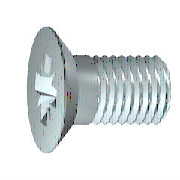
# Autodesk Inventor part: NF EN ISO 7046-2 H - M3x4 - 8.8 - H1
Saved by Autodesk Inventor 2019 (Build 230136000, 136)
## iProperties
Created: 2018-01-05
Part Number: NF EN ISO 7046-2 H - M3x4 - 8.8 - H1
Material: Acier inoxydable 440C
Description: Vis à tête fraisée plate (type de tête standard) avec empreinte cruciforme de type H ou Z
Document SubType Name: Modeling
Standard: NF EN ISO 7046-2 H
Designer: Sébastien DI MERCURIO
Standards Organization: AFNOR
Language: fr-FR
Size Designation: M3x4 - 8.8 - H1
Categories: <MemberInstance><Categories><Category DisplayName="Visserie" InternalName="e4da775c-781d-43d5-af7c-5136215cf5a6" Mnemonic="FSTN"><Category DisplayName="Vis" InternalName="536e6df0-f778-49ac-b2f2-25c71d2aa0b2" Mnemonic="SCRW"><CategoryParameter DisplayName="Désignation du diamètre nominal" InternalName="03caf894-eafd-4c09-a035-916ac084b87b" Mnemonic="nomdiadesig"/><CategoryParameter DisplayName="Longueur nominale" InternalName="238ecbaf-3e6c-45dd-aa95-4068c8e0fd02" Mnemonic="nomlen"/><CategoryParameter DisplayName="Désignation du filetage" InternalName="586d5e89-370a-4089-914f-0110033585c7" Mnemonic="thrdesign"/><CategoryParameter DisplayName="Désignation de série de filetage" InternalName="87c5849c-b3a5-4c3e-9c9b-2feecef9be86" Mnemonic="thrserdsgn"/><CategoryParameter DisplayName="Diamètre nominal" InternalName="8bbe3f8e-44cf-40a9-a251-3a6edc8168d6" Mnemonic="nomdia"/><CategoryParameter DisplayName="Type de taraudage" InternalName="b4bbb7bc-d6aa-4c9f-a9a9-4152b9f6fe49" Mnemonic="thrtype"/><CategoryParameter DisplayName="Pas de filetage" InternalName="bb82302e-82d8-4176-8fc1-c5d7bb17d5ad" Mnemonic="pitch1"/><CategoryParameter DisplayName="Filets par unité" InternalName="bdc6e7d2-ffd0-4d9c-a173-16b95ebb912d" Mnemonic="thrperunit1"/><CategoryParameter DisplayName="Classe de filetage" InternalName="ebc0d23b-2cc6-4d2a-b376-d52aae53bab6" Mnemonic="thrclss"/><Category DisplayName="Tête fraisée" InternalName="49656530-5684-4604-a233-68d537625f23" Mnemonic="CSSCRW"><CategoryParameter DisplayName="Type" InternalName="161b33bb-bee3-4fab-a17d-97511dff40f0" Mnemonic="type"/><CategoryParameter DisplayName="Longueur de filetage" InternalName="207f0278-6dec-43ab-bffc-1c6d03e64de4" Mnemonic="thrlen"/><CategoryParameter DisplayName="Longueur de serrage" InternalName="2fff3de5-ce2a-45fd-9425-99ddc9dff352" Mnemonic="grplen"/><CategoryParameter DisplayName="Classe de propriétés" InternalName="5249b721-5ecc-4781-a2e8-d7e3bda3ecca" Mnemonic="propclss"/><CategoryParameter DisplayName="Hauteur de tête" InternalName="57526df9-da71-45fb-acb4-1d0529a34778" Mnemonic="headh"/><CategoryParameter DisplayName="Diamètre de tige" InternalName="7ece923f-d8ee-40d5-83f8-980cad520964" Mnemonic="grpdia"/><CategoryParameter DisplayName="Diamètre de tête" InternalName="a509cd31-06d1-44c5-b54e-d7a695352906" Mnemonic="headdia"/><CategoryParameter DisplayName="Angle de tête" InternalName="dbcfc1e0-7990-403e-bc2e-90d1c639222a" Mnemonic="headang"/></Category></Category></Category><Category DisplayName="Type de données" InternalName="23b78d0f-2648-40c6-8793-ca6db495c9e8" Mnemonic="DATATYPE"><CategoryParameter DisplayName="AfficherNom" InternalName="05415f3d-3907-474b-a020-eb9d644f4cf3" Mnemonic="DISPLAYNAME"/><CategoryParameter DisplayName="Norme" InternalName="0c0a119c-1e12-4c84-803f-101930972f5e" Mnemonic="STANDARD"/><CategoryParameter DisplayName="Description" InternalName="13903e3d-64b1-4950-80da-f627842ea37f" Mnemonic="DESCRIPTION"/><CategoryParameter DisplayName="Désignation" InternalName="2675968c-4ce5-49e0-a4f5-552d29089031" Mnemonic="DESIGNATION"/><CategoryParameter DisplayName="Ligne par défaut" InternalName="2af9ec52-faaa-4026-b378-f9fa4afca842" Mnemonic="DEFAULTROW"/><CategoryParameter DisplayName="Nom de dossier" InternalName="3f06958e-8713-4116-9be7-ed6184ecc97b" Mnemonic="FOLDERNAME"/><CategoryParameter DisplayName="Guide révision" InternalName="45a75005-10b1-4dfc-8d6d-dfe629f0b93c" Mnemonic="REVISIONGUID"/><CategoryParameter DisplayName="NomFichier" InternalName="8b46a4cc-9585-4fed-90c3-899f57e09a73" Mnemonic="FILENAME"/><CategoryParameter DisplayName="OrgNorm" InternalName="8f5914e1-4693-403f-8ab5-d37768198c9d" Mnemonic="STDSORG"/><CategoryParameter DisplayName="Version de la famille" InternalName="914462f6-6e19-4b14-ba84-155b9680b1d0" Mnemonic="FAMILYREVISION"/><CategoryParameter DisplayName="Version standard" InternalName="91d5a463-65c2-4fde-b823-3b7fea5e8e17" Mnemonic="STANDARDREVISION"/><CategoryParameter DisplayName="Révision de membre" InternalName="a65d44b9-392f-4f4f-857b-e4b3d54996fe" Mnemonic="MEMBERREVISION"/><CategoryParameter DisplayName="DélimiterFormat" InternalName="bc51e27b-3422-4e78-93ef-cec197ddf230" Mnemonic="CLIPFORMAT"/><CategoryParameter DisplayName="Fabricant" InternalName="cd6c7a72-a28a-4e50-99a9-2c7f4e13e5ad" Mnemonic="MANUFACTURER"/><CategoryParameter DisplayName="NomInterne" InternalName="cf1d0246-76d9-4b4a-8305-fa0409afb5c1" Mnemonic="INTERNALNAME"/><CategoryParameter DisplayName="Métrique" InternalName="e2385c5b-1ea4-4823-96a8-8de651266ec3" Mnemonic="ISMETRIC"/><Category DisplayName="Pièce" InternalName="c0e0b642-3bcb-4cc8-9e80-f96d35c4afa4" Mnemonic="PART"><CategoryParameter DisplayName="Numéro de pièce" InternalName="016b6077-bfbe-49bd-92c9-d8d59c39c941" Mnemonic="PARTNUMBER"/><CategoryParameter DisplayName="Numéro de stock" InternalName="4dba7c1c-e26c-444e-836c-b08b433409a8" Mnemonic="STOCKNUMBER"/><CategoryParameter DisplayName="Clé matière" InternalName="5c9a8adb-dd2b-4535-b97f-0a94a95fe41f" Mnemonic="MATERIALKEY"/><CategoryParameter DisplayName="Matière" InternalName="818a152a-d3c3-49ca-80ee-df7d91421b8e" Mnemonic="MATERIAL"/></Category></Category><Category DisplayName="Carte héritée DA" InternalName="924fff40-ddd0-4eff-ad42-30e3774ef79e" Mnemonic="LEGACYMAPDA"><CategoryParameter DisplayName="CookieDA" InternalName="316934ee-8fe1-4c7a-9c36-f2d79e1add1a" Mnemonic="DACOOKIE"/></Category></Categories><FamilyTemplate Id="i7046h3"><FamilyTemplateParameters><FamilyTemplateParameter ObjectType="kUserParameterObject" ValueType="xs:double" Id="1" ObjectReferenceKey="NND"/><FamilyTemplateParameter ObjectType="kUserParameterObject" ValueType="xs:double" Id="2" ObjectReferenceKey="NLG"/><FamilyTemplateParameter ObjectType="kUserParameterObject" ValueType="xs:double" Id="3" ObjectReferenceKey="PTC"/><FamilyTemplateParameter ObjectType="kUserParameterObject" ValueType="xs:double" Id="4" ObjectReferenceKey="Dh"/><FamilyTemplateParameter ObjectType="kUserParameterObject" ValueType="xs:double" Id="5" ObjectReferenceKey="ParK"/><FamilyTemplateParameter ObjectType="kUserParameterObject" ValueType="xs:double" Id="7" ObjectReferenceKey="r"/><FamilyTemplateParameter ObjectType="kUserParameterObject" ValueType="xs:double" Id="9" ObjectReferenceKey="ParA"/><FamilyTemplateParameter ObjectType="kUserParameterObject" ValueType="xs:double" Id="11" ObjectReferenceKey="M"/><FamilyTemplateParameter ObjectType="kUserParameterObject" ValueType="xs:double" Id="118" ObjectReferenceKey="THREADDIA"/><FamilyTemplateParameter ObjectType="kUserParameterObject" ValueType="xs:string" Id="119" ObjectReferenceKey="TEMPLATE"/><FamilyTemplateParameter ObjectType="kPropertyObject" ValueType="xs:string" Id="100" ObjectReferenceKey="{32853F0F-3444-11d1-9E93-0060B03C1CA6}" SubObjectId="52"/><FamilyTemplateParameter ObjectType="kPropertyObject" ValueType="xs:string" Id="105" ObjectReferenceKey="{32853F0F-3444-11d1-9E93-0060B03C1CA6}" SubObjectId="5"/><FamilyTemplateParameter ObjectType="kPartComponentDefinitionObject" ValueType="xs:string" Id="110" SubObjectId="Material"/><FamilyTemplateParameter ObjectType="kThreadFeatureObject" ValueType="xs:structure" Id="300" ObjectReferenceKey="1002000010000000070c0000000000008000000000000000" SubObjectId="ThreadInfo"><FamilyTemplateParameter ObjectType="" ValueType="xs:string" Id="301" SubObjectId="ThreadDesignation"/><FamilyTemplateParameter ObjectType="" ValueType="xs:string" Id="302" SubObjectId="ThreadType"/><FamilyTemplateParameter ObjectType="" ValueType="xs:string" Id="303" SubObjectId="ThreadClass"/></FamilyTemplateParameter></FamilyTemplateParameters></FamilyTemplate><CategoryParameterMap><ParamToTemplateMap><ParamToTemplate CategoryParameter="//CategoryParameter[@InternalName='05415f3d-3907-474b-a020-eb9d644f4cf3']" ConstantValue="NF EN ISO 7046-2 H"/><ParamToTemplate CategoryParameter="//CategoryParameter[@InternalName='cf1d0246-76d9-4b4a-8305-fa0409afb5c1']" ConstantValue="B27BD451-F53C-4D36-8893-BAC8912BD1CB"/><ParamToTemplate CategoryParameter="//CategoryParameter[@InternalName='3f06958e-8713-4116-9be7-ed6184ecc97b']" ConstantValue="NF EN ISO 7046-2 H"/><ParamToTemplate CategoryParameter="//CategoryParameter[@InternalName='914462f6-6e19-4b14-ba84-155b9680b1d0']" ConstantValue="10"/><ParamToTemplate CategoryParameter="//CategoryParameter[@InternalName='bc51e27b-3422-4e78-93ef-cec197ddf230']" ConstantValue="CF_INVENTOR.STDPARTS"/><ParamToTemplate CategoryParameter="//CategoryParameter[@InternalName='e2385c5b-1ea4-4823-96a8-8de651266ec3']" ConstantValue="true"/><ParamToTemplate CategoryParameter="//CategoryParameter[@InternalName='13903e3d-64b1-4950-80da-f627842ea37f']" ConstantValue="Countersunk flat head screws (common head style) with type H or type Z cross recess."/><ParamToTemplate CategoryParameter="//CategoryParameter[@InternalName='8f5914e1-4693-403f-8ab5-d37768198c9d']" ConstantValue="AFNOR"/><ParamToTemplate CategoryParameter="//CategoryParameter[@InternalName='0c0a119c-1e12-4c84-803f-101930972f5e']" ConstantValue="NF EN ISO 7046-2 H"/><ParamToTemplate CategoryParameter="//CategoryParameter[@InternalName='cd6c7a72-a28a-4e50-99a9-2c7f4e13e5ad']" TemplateParameter="104"/><ParamToTemplate CategoryParameter="//CategoryParameter[@InternalName='91d5a463-65c2-4fde-b823-3b7fea5e8e17']" TemplateParameter="103"/><ParamToTemplate CategoryParameter="//CategoryParameter[@InternalName='45a75005-10b1-4dfc-8d6d-dfe629f0b93c']" ConstantValue="88fd80a9-c19a-4586-a11f-2e24e520522a"/><ParamToTemplate CategoryParameter="//CategoryParameter[@InternalName='2af9ec52-faaa-4026-b378-f9fa4afca842']" ConstantValue="10"/><ParamToTemplate CategoryParameter="//CategoryParameter[@InternalName='8b46a4cc-9585-4fed-90c3-899f57e09a73']" ConstantValue="NF EN ISO 7046-2 H - M3x4 - 8.8 - H1"/><ParamToTemplate CategoryParameter="//CategoryParameter[@InternalName='a65d44b9-392f-4f4f-857b-e4b3d54996fe']" ConstantValue="eb5f4cae-6e3a-428d-b8ef-d14df2735137"/><ParamToTemplate CategoryParameter="//CategoryParameter[@InternalName='2fff3de5-ce2a-45fd-9425-99ddc9dff352']" ConstantValue="1,25"/><ParamToTemplate CategoryParameter="//CategoryParameter[@InternalName='dbcfc1e0-7990-403e-bc2e-90d1c639222a']" ConstantValue="90"/><ParamToTemplate CategoryParameter="//CategoryParameter[@InternalName='03caf894-eafd-4c09-a035-916ac084b87b']" ConstantValue="M3"/><ParamToTemplate CategoryParameter="//CategoryParameter[@InternalName='316934ee-8fe1-4c7a-9c36-f2d79e1add1a']" ConstantValue="*AFN~I70462H~M3x4 - 8.8 - H1~4*"/><ParamToTemplate CategoryParameter="//CategoryParameter[@InternalName='2675968c-4ce5-49e0-a4f5-552d29089031']" TemplateParameter="100"/><ParamToTemplate CategoryParameter="//CategoryParameter[@InternalName='a509cd31-06d1-44c5-b54e-d7a695352906']" TemplateParameter="4"/><ParamToTemplate CategoryParameter="//CategoryParameter[@InternalName='818a152a-d3c3-49ca-80ee-df7d91421b8e']" TemplateParameter="110"/><ParamToTemplate CategoryParameter="//CategoryParameter[@InternalName='238ecbaf-3e6c-45dd-aa95-4068c8e0fd02']" TemplateParameter="2"/><ParamToTemplate CategoryParameter="//CategoryParameter[@InternalName='8bbe3f8e-44cf-40a9-a251-3a6edc8168d6']" TemplateParameter="1"/><ParamToTemplate CategoryParameter="//CategoryParameter[@InternalName='016b6077-bfbe-49bd-92c9-d8d59c39c941']" TemplateParameter="105"/><ParamToTemplate CategoryParameter="//CategoryParameter[@InternalName='bb82302e-82d8-4176-8fc1-c5d7bb17d5ad']" TemplateParameter="3"/><ParamToTemplate CategoryParameter="//CategoryParameter[@InternalName='57526df9-da71-45fb-acb4-1d0529a34778']" TemplateParameter="5"/><ParamToTemplate CategoryParameter="//CategoryParameter[@InternalName='ebc0d23b-2cc6-4d2a-b376-d52aae53bab6']" TemplateParameter="303"/><ParamToTemplate CategoryParameter="//CategoryParameter[@InternalName='586d5e89-370a-4089-914f-0110033585c7']" TemplateParameter="301"/><ParamToTemplate CategoryParameter="//CategoryParameter[@InternalName='b4bbb7bc-d6aa-4c9f-a9a9-4152b9f6fe49']" TemplateParameter="302"/><ParamToTemplate CategoryParameter="//CategoryParameter[@InternalName='207f0278-6dec-43ab-bffc-1c6d03e64de4']" TemplateParameter="8"/></ParamToTemplateMap></CategoryParameterMap></MemberInstance>
Density: 7.75 g/cm^3
Appearance: Semi-poli
IsCustomPart: 0
Author: Sébastien DI MERCURIO
Autodesk Inventor part; units mm, degrees
ref_plane "YZ Plane" through (0, 0, 0) normal (1, 0, 0) x (0, 1, 0)
sketch "Esquisse1" plane through (0, 0, 0) normal (0, 1, 0) x (-1, 0, 0)
  point P0 (0, 0)
sketch "Esquisse2" plane through (0, 0, 0) normal (0, 0, 1) x (1, 0, 0)
  point P0 (0, 0)
sketch "Esquisse3" plane through (0, 0, 0) normal (0, 0, 1) x (1, 0, 0)
  point P0 (0, 0)
sketch "Esquisse4" plane through (0, 0, 0) normal (0, 1, 0) x (-1, 0, 0)
  line L0 (-2.75, 0) -> (0, 0)
  line L1 (-2.75, -0.4) -> (-2.75, 0)
  line L2 (-1.5, -1.65) -> (-2.75, -0.4)
  line L3 (-1.5, -1.9) -> (-1.5, -1.65)
  line L4 (-1.25, -2.15) -> (-1.5, -1.9)
  line L5 (-1.5, -2.4) -> (-1.25, -2.15)
  line L6 (-1.5, -4) -> (-1.5, -2.4)
  line L7 (0, 0) -> (0, -4)
  line L8 (0, 3.3392) -> (0, -10.7) construction
  line L9 (0, 3.3392) -> (0, -10.7)
  line L10 (0, -13.5078) -> (0, 6.1471) projected
  line L11 (-1.5, -4) -> (0, -4)
  line L12 (0.55, 0) -> (-3.3, 0) projected
  dimension "d3" = 2.75
  dimension "d5" = 0.25
  dimension "d7" = 0.25
  dimension "d9" = 0.25
  dimension "d11" = 1.65
  dimension "d13" = 135
  dimension "d17" = 1.25
  dimension "d19" = 0
  dimension "d51" = 1.5
  dimension "d52" = 4
  constraints: 22 end point, 5 vertical, 3 collinear, 1 horizontal, 1 perpendicular
  measures "d3" distance of L0.start L0.end
  measures "d5" horizontal distance of L5.start L4.start
  measures "d7" horizontal distance of L4.start L3.start
  measures "d9" distance of L3.start L2.start
  measures "d11" vertical distance of L2.start L0.start
  measures "d13" angle of L3 L2
  measures "d17" horizontal distance of L4.start L0.end
  measures "d19" horizontal distance of L8.start L0.end
  measures "d51" distance of L6.start L7.end
  measures "d52" distance between parallel lines of L11 L0
revolve "Révolution1" add sketch "Esquisse4" angle 360 about axis through (0, 0, 3.3392) along (0, 0, -1)
sketch "Esquisse5" plane through (0, 0, 0) normal (0, 1, 0) x (-1, 0, 0)
  line L0 (-1.6, 0) -> (0, 0)
  line L1 (-0.2667, -1.5) -> (-1.6, 0)
  line L2 (0, -1.5) -> (-0.2667, -1.5)
  line L3 (0, 0) -> (0, -1.5)
  line L4 (-1.5, -1.65) -> (1.5, -1.65) construction
  line L5 (-2.75, 0) -> (2.75, 0) projected
  line L6 (0, -1.98) -> (0, 0.33) projected
  dimension "d22" = 1.6
  dimension "d24" = 0.2667
  dimension "d26" = 1.5
  constraints: 8 end point, 2 collinear, 2 horizontal, 1 vertical
  measures "d22" distance of L0.start L0.end
  measures "d24" distance of L2.start L1.start
  measures "d26" distance of L0.end L2.start
extrude "Extrusion1" cut sketch "Esquisse5" along normal mid plane 0.5333
pattern_circular "RéseauPolaire1" count 4 over 360 about axis through (0, 0, 0) along (0, 0, 1) of "Extrusion1"
sketch "Esquisse7" plane through (0, 0, 0) normal (0, 1, 0) x (-1, 0, 0)
  line L0 (0, -0.825) -> (-2, 0)
  line L1 (0, 0) -> (0, -0.825)
  line L2 (-2, 0) -> (0, 0)
  line L3 (-1.5, -1.65) -> (1.5, -1.65) construction
  line L4 (0, -1.98) -> (0, 0.33) projected
  line L5 (-2.75, 0) -> (2.75, 0) projected
  dimension "d33" = 2
  dimension "d35" = 0.825
  constraints: 6 end point, 2 collinear, 1 horizontal, 1 vertical
  measures "d33" distance of L0.end L1.start
  measures "d35" distance of L1.start L0.start
extrude "Extrusion2" cut sketch "Esquisse7" along normal mid plane 0.5333
pattern_circular "RéseauPolaire2" count 4 over 360 about axis through (0, 0, 0) along (0, 0, 1) of "Extrusion2"
fillet "Congé1" radius 0.5 1 edges at (-1.5, 0, -1.65)
thread "Filetage1" size "M3x0.5" class "6g" standard "ISO Metric profile" full length
ref_plane "MSC_PF1" through (0, 0, 0) normal (1, 0, 0) x (0, 1, 0)
ref_plane "MSC_PT1" through (0, 0, 0) normal (0, 0, -1) x (-1, 0, 0)
equation "\"d3\" = 0.5 * Dh"
equation "\"d5\" = msp_x"
equation "\"d7\" = ParA"
equation "\"d9\" = msp_x"
equation "\"d11\" = ParK"
equation "\"d17\" = 0.5 * msp_mdtds"
equation "\"d51\" = 0.5 * NND"
equation "\"d52\" = NLG"
equation "\"d22\" = 0.5 * M"
equation "\"d24\" = 0.0833333 * M"
equation "\"d26\" = 0.909091 * ParK"
equation "\"d27\" = 0.166667 * M"
equation "\"d33\" = 0.625 * M"
equation "\"d35\" = 0.5 * ParK"
equation "\"d36\" = 0.166667 * M"
equation "\"d41\" = 2 * msp_x"
equation "\"PTC\" = 0.5"
equation "\"NLG\" = 4"
equation "\"ParK\" = 1.65"
equation "\"NND\" = 3"
equation "\"M\" = 3.2"
equation "\"msp_mdtds\" = NND - PTC"
equation "\"Dh\" = 5.5"
equation "\"msp_x\" = 0.5 * PTC"
equation "\"ParA\" = 0.5 * PTC"
equation "\"r\" = 0.8"
equation "\"THREADDIA\" = NND"
equation "\"TEMPLATE\" = 1.2345"
body "Solid1"
